Autodesk Fusion 360 part; units mm, degrees
(part 11 of 12)
  line L934 (66.0376, -20.82) -> (65.7437, -20.7245)
  line L935 (66.0427, -20.82) -> (66.0376, -20.82)
  line L936 (65.7437, -19.9155) -> (66.0376, -19.82)
  line L937 (66.5182, -20.4745) -> (66.3366, -20.7245)
  line L938 (65.5621, -20.1655) -> (65.7437, -19.9155)
  line L939 (66.5182, -20.1655) -> (66.5182, -20.4745)
  line L940 (66.0427, -19.82) -> (66.3366, -19.9155)
  line L941 (65.5621, -20.4745) -> (65.5621, -20.1655)
  line L942 (65.7437, -20.7245) -> (65.5621, -20.4745)
  line L943 (65.7437, -22.4555) -> (66.0376, -22.36)
  line L944 (66.3366, -22.4555) -> (66.5182, -22.7055)
  line L945 (66.5182, -23.0146) -> (66.3366, -23.2646)
  line L946 (66.0427, -22.36) -> (66.3366, -22.4555)
  line L947 (65.7437, -23.2646) -> (65.5621, -23.0146)
  line L948 (66.5182, -22.7055) -> (66.5182, -23.0146)
  line L949 (65.5621, -23.0146) -> (65.5621, -22.7055)
  line L950 (66.3366, -23.2646) -> (66.0427, -23.36)
  line L951 (66.0376, -23.36) -> (65.7437, -23.2646)
  line L952 (66.0427, -23.36) -> (66.0376, -23.36)
  line L953 (65.5621, -22.7055) -> (65.7437, -22.4555)
  line L954 (66.0376, -22.36) -> (66.0427, -22.36)
  line L955 (84.2982, -22.7055) -> (84.2982, -23.0146)
  line L956 (84.2982, -23.0146) -> (84.1166, -23.2646)
  line L957 (84.1166, -22.4555) -> (84.2982, -22.7055)
  line L958 (83.3421, -23.0146) -> (83.3421, -22.7055)
  line L959 (83.8227, -23.36) -> (83.8176, -23.36)
  line L960 (83.5237, -23.2646) -> (83.3421, -23.0146)
  line L961 (83.8227, -22.36) -> (84.1166, -22.4555)
  line L962 (83.8176, -23.36) -> (83.5237, -23.2646)
  line L963 (84.1166, -23.2646) -> (83.8227, -23.36)
  line L964 (83.5237, -22.4555) -> (83.8176, -22.36)
  line L965 (83.8176, -22.36) -> (83.8227, -22.36)
  line L966 (83.3421, -22.7055) -> (83.5237, -22.4555)
  line L967 (83.8176, -19.82) -> (83.8227, -19.82)
  line L968 (84.1166, -20.7245) -> (83.8227, -20.82)
  line L969 (83.8227, -19.82) -> (84.1166, -19.9155)
  line L970 (83.5237, -19.9155) -> (83.8176, -19.82)
  line L971 (84.1166, -19.9155) -> (84.2982, -20.1655)
  line L972 (84.2982, -20.4745) -> (84.1166, -20.7245)
  line L973 (83.3421, -20.4745) -> (83.3421, -20.1655)
  line L974 (84.2982, -20.1655) -> (84.2982, -20.4745)
  line L975 (83.5237, -20.7245) -> (83.3421, -20.4745)
  line L976 (83.8227, -20.82) -> (83.8176, -20.82)
  line L977 (83.8176, -20.82) -> (83.5237, -20.7245)
  line L978 (83.3421, -20.1655) -> (83.5237, -19.9155)
  line L979 (84.2982, -18.0062) -> (84.1166, -18.2562)
  line L980 (83.3421, -17.6972) -> (83.5237, -17.4472)
  line L981 (84.1166, -18.2562) -> (83.8227, -18.3517)
  line L982 (83.8227, -17.3517) -> (84.1166, -17.4472)
  line L983 (84.2982, -17.6972) -> (84.2982, -18.0062)
  line L984 (83.5237, -17.4472) -> (83.8176, -17.3517)
  line L985 (83.8176, -17.3517) -> (83.8227, -17.3517)
  line L986 (83.8227, -18.3517) -> (83.8176, -18.3517)
  line L987 (83.3421, -18.0062) -> (83.3421, -17.6972)
  line L988 (84.1166, -17.4472) -> (84.2982, -17.6972)
  line L989 (83.5237, -18.2562) -> (83.3421, -18.0062)
  line L990 (83.8176, -18.3517) -> (83.5237, -18.2562)
  line L991 (83.8176, -15.74) -> (83.5237, -15.6445)
  line L992 (84.2982, -15.0855) -> (84.2982, -15.3945)
  line L993 (83.8176, -14.74) -> (83.8227, -14.74)
  line L994 (83.8227, -14.74) -> (84.1166, -14.8355)
  line L995 (84.1166, -14.8355) -> (84.2982, -15.0855)
  line L996 (84.1166, -15.6445) -> (83.8227, -15.74)
  line L997 (84.2982, -15.3945) -> (84.1166, -15.6445)
  line L998 (83.3421, -15.0855) -> (83.5237, -14.8355)
  line L999 (83.5237, -15.6445) -> (83.3421, -15.3945)
  line L1000 (83.8227, -15.74) -> (83.8176, -15.74)
  line L1001 (83.3421, -15.3945) -> (83.3421, -15.0855)
  line L1002 (83.5237, -14.8355) -> (83.8176, -14.74)
  line L1003 (83.8176, -12.2) -> (83.8227, -12.2)
  line L1004 (83.5237, -12.2955) -> (83.8176, -12.2)
  line L1005 (83.8176, -13.2) -> (83.5237, -13.1045)
  line L1006 (84.1166, -13.1045) -> (83.8227, -13.2)
  line L1007 (83.8227, -13.2) -> (83.8176, -13.2)
  line L1008 (84.2982, -12.5455) -> (84.2982, -12.8545)
  line L1009 (83.8227, -12.2) -> (84.1166, -12.2955)
  line L1010 (84.1166, -12.2955) -> (84.2982, -12.5455)
  line L1011 (83.3421, -12.5455) -> (83.5237, -12.2955)
  line L1012 (84.2982, -12.8545) -> (84.1166, -13.1045)
  line L1013 (83.5237, -13.1045) -> (83.3421, -12.8545)
  line L1014 (83.3421, -12.8545) -> (83.3421, -12.5455)
  line L1015 (84.1166, -10.5645) -> (83.8227, -10.66)
  line L1016 (84.1166, -9.7555) -> (84.2982, -10.0055)
  line L1017 (83.8227, -9.66) -> (84.1166, -9.7555)
  line L1018 (83.5237, -9.7555) -> (83.8176, -9.66)
  line L1019 (84.2982, -10.0055) -> (84.2982, -10.3145)
  line L1020 (83.3421, -10.3145) -> (83.3421, -10.0055)
  line L1021 (83.8176, -9.66) -> (83.8227, -9.66)
  line L1022 (83.3421, -10.0055) -> (83.5237, -9.7555)
  line L1023 (83.8176, -10.66) -> (83.5237, -10.5645)
  line L1024 (83.5237, -10.5645) -> (83.3421, -10.3145)
  line L1025 (83.8227, -10.66) -> (83.8176, -10.66)
  line L1026 (84.2982, -10.3145) -> (84.1166, -10.5645)
  line L1027 (83.8176, -8.12) -> (83.5237, -8.0245)
  line L1028 (83.8227, -7.12) -> (84.1166, -7.2155)
  line L1029 (83.3421, -7.4655) -> (83.5237, -7.2155)
  line L1030 (83.8176, -7.12) -> (83.8227, -7.12)
  line L1031 (83.5237, -7.2155) -> (83.8176, -7.12)
  line L1032 (84.2982, -7.7745) -> (84.1166, -8.0245)
  line L1033 (83.8227, -8.12) -> (83.8176, -8.12)
  line L1034 (84.2982, -7.4655) -> (84.2982, -7.7745)
  line L1035 (83.3421, -7.7745) -> (83.3421, -7.4655)
  line L1036 (83.5237, -8.0245) -> (83.3421, -7.7745)
  line L1037 (84.1166, -7.2155) -> (84.2982, -7.4655)
  line L1038 (84.1166, -8.0245) -> (83.8227, -8.12)
  line L1039 (83.5237, -4.6755) -> (83.8176, -4.58)
  line L1040 (84.1166, -5.4845) -> (83.8227, -5.58)
  line L1041 (83.8227, -4.58) -> (84.1166, -4.6755)
  line L1042 (84.2982, -4.9255) -> (84.2982, -5.2345)
  line L1043 (84.1166, -4.6755) -> (84.2982, -4.9255)
  line L1044 (83.5237, -5.4845) -> (83.3421, -5.2345)
  line L1045 (83.3421, -5.2345) -> (83.3421, -4.9255)
  line L1046 (83.8176, -5.58) -> (83.5237, -5.4845)
  line L1047 (83.8176, -4.58) -> (83.8227, -4.58)
  line L1048 (83.3421, -4.9255) -> (83.5237, -4.6755)
  line L1049 (83.8227, -5.58) -> (83.8176, -5.58)
  line L1050 (84.2982, -5.2345) -> (84.1166, -5.4845)
  line L1051 (84.2982, -2.3855) -> (84.2982, -2.6945)
  line L1052 (83.5237, -2.1355) -> (83.8176, -2.04)
  line L1053 (83.5237, -2.9445) -> (83.3421, -2.6945)
  line L1054 (84.1166, -2.1355) -> (84.2982, -2.3855)
  line L1055 (83.8176, -2.04) -> (83.8227, -2.04)
  line L1056 (83.3421, -2.6945) -> (83.3421, -2.3855)
  line L1057 (83.8227, -2.04) -> (84.1166, -2.1355)
  line L1058 (83.8227, -3.04) -> (83.8176, -3.04)
  line L1059 (83.3421, -2.3855) -> (83.5237, -2.1355)
  line L1060 (83.8176, -3.04) -> (83.5237, -2.9445)
  line L1061 (84.1166, -2.9445) -> (83.8227, -3.04)
  line L1062 (84.2982, -2.6945) -> (84.1166, -2.9445)
  line L1063 (83.8176, -0.5) -> (83.5237, -0.4045)
  line L1064 (83.5237, 0.4045) -> (83.8176, 0.5)
  line L1065 (83.8176, 0.5) -> (83.8227, 0.5)
  line L1066 (83.5237, -0.4045) -> (83.3421, -0.1545)
  line L1067 (84.2982, 0.1545) -> (84.2982, -0.1545)
  line L1068 (84.1166, -0.4045) -> (83.8227, -0.5)
  line L1069 (83.3421, -0.1545) -> (83.3421, 0.1545)
  line L1070 (83.3421, 0.1545) -> (83.5237, 0.4045)
  line L1071 (83.8227, 0.5) -> (84.1166, 0.4045)
  line L1072 (83.8227, -0.5) -> (83.8176, -0.5)
  line L1073 (84.1166, 0.4045) -> (84.2982, 0.1545)
  line L1074 (84.2982, -0.1545) -> (84.1166, -0.4045)
  line L1075 (84.1166, 2.9445) -> (84.2982, 2.6945)
  line L1076 (83.5237, 2.1355) -> (83.3421, 2.3855)
  line L1077 (83.8227, 2.04) -> (83.8176, 2.04)
  line L1078 (84.2982, 2.6945) -> (84.2982, 2.3855)
  line L1079 (83.8227, 3.04) -> (84.1166, 2.9445)
  line L1080 (83.3421, 2.3855) -> (83.3421, 2.6945)
  line L1081 (83.8176, 3.04) -> (83.8227, 3.04)
  line L1082 (83.5237, 2.9445) -> (83.8176, 3.04)
  line L1083 (83.8176, 2.04) -> (83.5237, 2.1355)
  line L1084 (83.3421, 2.6945) -> (83.5237, 2.9445)
  line L1085 (84.2982, 2.3855) -> (84.1166, 2.1355)
  line L1086 (84.1166, 2.1355) -> (83.8227, 2.04)
  line L1087 (83.5237, 4.6755) -> (83.3421, 4.9255)
  line L1088 (83.3421, 4.9255) -> (83.3421, 5.2345)
  line L1089 (83.5237, 5.4845) -> (83.8176, 5.58)
  line L1090 (84.2982, 4.9255) -> (84.1166, 4.6755)
  line L1091 (83.8176, 5.58) -> (83.8227, 5.58)
  line L1092 (84.1166, 5.4845) -> (84.2982, 5.2345)
  line L1093 (84.1166, 4.6755) -> (83.8227, 4.58)
  line L1094 (83.3421, 5.2345) -> (83.5237, 5.4845)
  line L1095 (84.2982, 5.2345) -> (84.2982, 4.9255)
  line L1096 (83.8227, 5.58) -> (84.1166, 5.4845)
  line L1097 (83.8176, 4.58) -> (83.5237, 4.6755)
  line L1098 (83.8227, 4.58) -> (83.8176, 4.58)
  line L1099 (83.3421, 7.4655) -> (83.3421, 7.7745)
  line L1100 (83.3421, 7.7745) -> (83.5237, 8.0245)
  line L1101 (84.1166, 8.0245) -> (84.2982, 7.7745)
  line L1102 (83.5237, 8.0245) -> (83.8176, 8.12)
  line L1103 (83.8176, 7.12) -> (83.5237, 7.2155)
  line L1104 (84.2982, 7.4655) -> (84.1166, 7.2155)
  line L1105 (84.2982, 7.7745) -> (84.2982, 7.4655)
  line L1106 (83.5237, 7.2155) -> (83.3421, 7.4655)
  line L1107 (83.8176, 8.12) -> (83.8227, 8.12)
  line L1108 (83.8227, 8.12) -> (84.1166, 8.0245)
  line L1109 (83.8227, 7.12) -> (83.8176, 7.12)
  line L1110 (84.1166, 7.2155) -> (83.8227, 7.12)
  line L1111 (84.2982, 10.3145) -> (84.2982, 10.0055)
  line L1112 (83.8227, 10.66) -> (84.1166, 10.5645)
  line L1113 (83.8176, 10.66) -> (83.8227, 10.66)
  line L1114 (84.2982, 10.0055) -> (84.1166, 9.7555)
  line L1115 (83.3421, 10.0055) -> (83.3421, 10.3145)
  line L1116 (83.3421, 10.3145) -> (83.5237, 10.5645)
  line L1117 (83.8227, 9.66) -> (83.8176, 9.66)
  line L1118 (84.1166, 10.5645) -> (84.2982, 10.3145)
  line L1119 (83.5237, 9.7555) -> (83.3421, 10.0055)
  line L1120 (83.5237, 10.5645) -> (83.8176, 10.66)
  line L1121 (83.8176, 9.66) -> (83.5237, 9.7555)
  line L1122 (84.1166, 9.7555) -> (83.8227, 9.66)
  line L1123 (84.1166, 13.1045) -> (84.2982, 12.8545)
  line L1124 (83.3421, 12.8545) -> (83.5237, 13.1045)
  line L1125 (83.5237, 12.2955) -> (83.3421, 12.5455)
  line L1126 (83.8176, 12.2) -> (83.5237, 12.2955)
  line L1127 (83.3421, 12.5455) -> (83.3421, 12.8545)
  line L1128 (83.5237, 13.1045) -> (83.8176, 13.2)
  line L1129 (83.8227, 13.2) -> (84.1166, 13.1045)
  line L1130 (84.2982, 12.8545) -> (84.2982, 12.5455)
  line L1131 (84.1166, 12.2955) -> (83.8227, 12.2)
  line L1132 (84.2982, 12.5455) -> (84.1166, 12.2955)
  line L1133 (83.8176, 13.2) -> (83.8227, 13.2)
  line L1134 (83.8227, 12.2) -> (83.8176, 12.2)
  line L1135 (83.3421, 15.0855) -> (83.3421, 15.3945)
  line L1136 (83.5237, 15.6445) -> (83.8176, 15.74)
  line L1137 (83.5237, 14.8355) -> (83.3421, 15.0855)
  line L1138 (84.2982, 15.0855) -> (84.1166, 14.8355)
  line L1139 (83.3421, 15.3945) -> (83.5237, 15.6445)
  line L1140 (84.2982, 15.3945) -> (84.2982, 15.0855)
  line L1141 (84.1166, 15.6445) -> (84.2982, 15.3945)
  line L1142 (84.1166, 14.8355) -> (83.8227, 14.74)
  line L1143 (83.8176, 15.74) -> (83.8227, 15.74)
  line L1144 (83.8227, 14.74) -> (83.8176, 14.74)
  line L1145 (83.8176, 14.74) -> (83.5237, 14.8355)
  line L1146 (83.8227, 15.74) -> (84.1166, 15.6445)
  line L1147 (83.5237, 17.3755) -> (83.3421, 17.6255)
  line L1148 (83.8227, 18.28) -> (84.1166, 18.1845)
  line L1149 (83.3421, 17.9345) -> (83.5237, 18.1845)
  line L1150 (84.2982, 17.6255) -> (84.1166, 17.3755)
  line L1151 (83.8176, 17.28) -> (83.5237, 17.3755)
  line L1152 (84.2982, 17.9345) -> (84.2982, 17.6255)
  line L1153 (83.3421, 17.6255) -> (83.3421, 17.9345)
  line L1154 (84.1166, 18.1845) -> (84.2982, 17.9345)
  line L1155 (83.5237, 18.1845) -> (83.8176, 18.28)
  line L1156 (84.1166, 17.3755) -> (83.8227, 17.28)
  line L1157 (83.8227, 17.28) -> (83.8176, 17.28)
  line L1158 (83.8176, 18.28) -> (83.8227, 18.28)
  line L1159 (83.8227, 19.82) -> (83.8176, 19.82)
  line L1160 (83.5237, 20.7245) -> (83.8176, 20.82)
  line L1161 (83.3421, 20.4745) -> (83.5237, 20.7245)
  line L1162 (84.1166, 20.7245) -> (84.2982, 20.4745)
  line L1163 (84.2982, 20.4745) -> (84.2982, 20.1655)
  line L1164 (83.5237, 19.9155) -> (83.3421, 20.1655)
  line L1165 (83.8227, 20.82) -> (84.1166, 20.7245)
  line L1166 (84.2982, 20.1655) -> (84.1166, 19.9155)
  line L1167 (83.3421, 20.1655) -> (83.3421, 20.4745)
  line L1168 (83.8176, 20.82) -> (83.8227, 20.82)
  line L1169 (84.1166, 19.9155) -> (83.8227, 19.82)
  line L1170 (83.8176, 19.82) -> (83.5237, 19.9155)
  line L1171 (84.2982, 22.7055) -> (84.1166, 22.4555)
  line L1172 (83.5237, 23.2646) -> (83.8176, 23.36)
  line L1173 (83.8176, 22.36) -> (83.5237, 22.4555)
  line L1174 (84.1166, 23.2646) -> (84.2982, 23.0146)
  line L1175 (83.3421, 23.0146) -> (83.5237, 23.2646)
  line L1176 (84.2982, 23.0146) -> (84.2982, 22.7055)
  line L1177 (83.8227, 23.36) -> (84.1166, 23.2646)
  line L1178 (83.8227, 22.36) -> (83.8176, 22.36)
  line L1179 (83.3421, 22.7055) -> (83.3421, 23.0146)
  line L1180 (83.8176, 23.36) -> (83.8227, 23.36)
  line L1181 (84.1166, 22.4555) -> (83.8227, 22.36)
  line L1182 (83.5237, 22.4555) -> (83.3421, 22.7055)
  line L1183 (83.5237, 25.8046) -> (83.8176, 25.9001)
  line L1184 (84.1166, 24.9955) -> (83.8227, 24.9001)
  line L1185 (83.8227, 24.9001) -> (83.8176, 24.9001)
  line L1186 (84.1166, 25.8046) -> (84.2982, 25.5546)
  line L1187 (83.3421, 25.5546) -> (83.5237, 25.8046)
  line L1188 (83.8176, 25.9001) -> (83.8227, 25.9001)
  line L1189 (83.8227, 25.9001) -> (84.1166, 25.8046)
  line L1190 (84.2982, 25.5546) -> (84.2982, 25.2455)
  line L1191 (83.3421, 25.2455) -> (83.3421, 25.5546)
  line L1192 (84.2982, 25.2455) -> (84.1166, 24.9955)
  line L1193 (83.8176, 24.9001) -> (83.5237, 24.9955)
  line L1194 (83.5237, 24.9955) -> (83.3421, 25.2455)
  line L1195 (70.8237, -23.2646) -> (70.6421, -23.0146)
  line L1196 (71.1176, -23.36) -> (70.8237, -23.2646)
  line L1197 (71.5982, -23.0146) -> (71.4166, -23.2646)
  line L1198 (70.8237, -22.4555) -> (71.1176, -22.36)
  line L1199 (71.5982, -22.7055) -> (71.5982, -23.0146)
  line L1200 (71.4166, -23.2646) -> (71.1227, -23.36)
  line L1201 (71.1176, -22.36) -> (71.1227, -22.36)
  line L1202 (71.1227, -23.36) -> (71.1176, -23.36)
  line L1203 (70.6421, -23.0146) -> (70.6421, -22.7055)
  line L1204 (71.1227, -22.36) -> (71.4166, -22.4555)
  line L1205 (70.6421, -22.7055) -> (70.8237, -22.4555)
  line L1206 (71.4166, -22.4555) -> (71.5982, -22.7055)
  line L1207 (74.1382, -23.0146) -> (73.9566, -23.2646)
  line L1208 (73.1821, -22.7055) -> (73.3637, -22.4555)
  line L1209 (73.9566, -22.4555) -> (74.1382, -22.7055)
  line L1210 (73.1821, -23.0146) -> (73.1821, -22.7055)
  line L1211 (73.6627, -22.36) -> (73.9566, -22.4555)
  line L1212 (73.6576, -22.36) -> (73.6627, -22.36)
  line L1213 (73.6576, -23.36) -> (73.3637, -23.2646)
  line L1214 (73.3637, -22.4555) -> (73.6576, -22.36)
  line L1215 (74.1382, -22.7055) -> (74.1382, -23.0146)
  line L1216 (73.3637, -23.2646) -> (73.1821, -23.0146)
  line L1217 (73.6627, -23.36) -> (73.6576, -23.36)
  line L1218 (73.9566, -23.2646) -> (73.6627, -23.36)
  line L1219 (76.4966, -22.4555) -> (76.6782, -22.7055)
  line L1220 (76.6782, -23.0146) -> (76.4966, -23.2646)
  line L1221 (76.6782, -22.7055) -> (76.6782, -23.0146)
  line L1222 (76.4966, -23.2646) -> (76.2027, -23.36)
  line L1223 (76.2027, -22.36) -> (76.4966, -22.4555)
  line L1224 (76.2027, -23.36) -> (76.1976, -23.36)
  line L1225 (76.1976, -22.36) -> (76.2027, -22.36)
  line L1226 (75.9037, -22.4555) -> (76.1976, -22.36)
  line L1227 (75.7221, -22.7055) -> (75.9037, -22.4555)
  line L1228 (75.7221, -23.0146) -> (75.7221, -22.7055)
  line L1229 (75.9037, -23.2646) -> (75.7221, -23.0146)
  line L1230 (76.1976, -23.36) -> (75.9037, -23.2646)
  line L1231 (78.7376, -23.36) -> (78.4437, -23.2646)
  line L1232 (78.7376, -22.36) -> (78.7427, -22.36)
  line L1233 (79.0366, -23.2646) -> (78.7427, -23.36)
  line L1234 (79.2182, -23.0146) -> (79.0366, -23.2646)
  line L1235 (78.7427, -23.36) -> (78.7376, -23.36)
  line L1236 (79.2182, -22.7055) -> (79.2182, -23.0146)
  line L1237 (78.4437, -23.2646) -> (78.2621, -23.0146)
  line L1238 (78.7427, -22.36) -> (79.0366, -22.4555)
  line L1239 (79.0366, -22.4555) -> (79.2182, -22.7055)
  line L1240 (78.4437, -22.4555) -> (78.7376, -22.36)
  line L1241 (78.2621, -23.0146) -> (78.2621, -22.7055)
  line L1242 (78.2621, -22.7055) -> (78.4437, -22.4555)
  arc A2166 (-180.75, 30) -> (-179.25, 30) centre (-180, 30) ccw
  arc A2167 (-179.25, 30) -> (-180.75, 30) centre (-180, 30) ccw
  arc A2168 (-185.588, 27.46) -> (-187.112, 27.46) centre (-186.35, 27.46) ccw
  arc A2169 (-187.112, 27.46) -> (-185.588, 27.46) centre (-186.35, 27.46) ccw
  arc A2170 (-149.25, 30) -> (-150.75, 30) centre (-150, 30) ccw
  arc A2171 (-150.75, 30) -> (-149.25, 30) centre (-150, 30) ccw
  arc A2172 (-157.112, 27.46) -> (-155.588, 27.46) centre (-156.35, 27.46) ccw
  arc A2173 (-155.588, 27.46) -> (-157.112, 27.46) centre (-156.35, 27.46) ccw
  arc A2174 (-120.75, 30) -> (-119.25, 30) centre (-120, 30) ccw
  arc A2175 (-119.25, 30) -> (-120.75, 30) centre (-120, 30) ccw
  arc A2176 (-127.112, 27.46) -> (-125.588, 27.46) centre (-126.35, 27.46) ccw
  arc A2177 (-125.588, 27.46) -> (-127.112, 27.46) centre (-126.35, 27.46) ccw
  arc A2178 (-90.75, 30) -> (-89.25, 30) centre (-90, 30) ccw
  arc A2179 (-89.25, 30) -> (-90.75, 30) centre (-90, 30) ccw
  arc A2180 (-97.112, 27.46) -> (-95.588, 27.46) centre (-96.35, 27.46) ccw
  arc A2181 (-95.588, 27.46) -> (-97.112, 27.46) centre (-96.35, 27.46) ccw
  arc A2182 (-60.75, 30) -> (-59.25, 30) centre (-60, 30) ccw
  arc A2183 (-59.25, 30) -> (-60.75, 30) centre (-60, 30) ccw
  arc A2184 (-65.588, 27.46) -> (-67.112, 27.46) centre (-66.35, 27.46) ccw
  arc A2185 (-67.112, 27.46) -> (-65.588, 27.46) centre (-66.35, 27.46) ccw
  arc A2186 (-30.75, 30) -> (-29.25, 30) centre (-30, 30) ccw
  arc A2187 (-29.25, 30) -> (-30.75, 30) centre (-30, 30) ccw
  arc A2188 (-37.112, 27.46) -> (-35.588, 27.46) centre (-36.35, 27.46) ccw
  arc A2189 (-35.588, 27.46) -> (-37.112, 27.46) centre (-36.35, 27.46) ccw
  arc A2190 (-0.75, 30) -> (0.75, 30) centre (0, 30) ccw
  arc A2191 (0.75, 30) -> (-0.75, 30) centre (0, 30) ccw
  arc A2192 (-5.588, 27.46) -> (-7.112, 27.46) centre (-6.35, 27.46) ccw
  arc A2193 (-7.112, 27.46) -> (-5.588, 27.46) centre (-6.35, 27.46) ccw
  arc A2194 (29.25, 30) -> (30.75, 30) centre (30, 30) ccw
  arc A2195 (30.75, 30) -> (29.25, 30) centre (30, 30) ccw
  arc A2196 (24.412, 27.46) -> (22.888, 27.46) centre (23.65, 27.46) ccw
  arc A2197 (22.888, 27.46) -> (24.412, 27.46) centre (23.65, 27.46) ccw
  arc A2198 (-180.75, 0) -> (-179.25, 0) centre (-180, 0) ccw
  arc A2199 (-179.25, 0) -> (-180.75, 0) centre (-180, 0) ccw
  arc A2200 (-187.112, -2.54) -> (-185.588, -2.54) centre (-186.35, -2.54) ccw
  arc A2201 (-185.588, -2.54) -> (-187.112, -2.54) centre (-186.35, -2.54) ccw
  arc A2202 (-149.25, 0) -> (-150.75, 0) centre (-150, 0) ccw
  arc A2203 (-150.75, 0) -> (-149.25, 0) centre (-150, 0) ccw
  arc A2204 (-157.112, -2.54) -> (-155.588, -2.54) centre (-156.35, -2.54) ccw
  arc A2205 (-155.588, -2.54) -> (-157.112, -2.54) centre (-156.35, -2.54) ccw
  arc A2206 (-120.75, 0) -> (-119.25, 0) centre (-120, 0) ccw
  arc A2207 (-119.25, 0) -> (-120.75, 0) centre (-120, 0) ccw
  arc A2208 (-127.112, -2.54) -> (-125.588, -2.54) centre (-126.35, -2.54) ccw
  arc A2209 (-125.588, -2.54) -> (-127.112, -2.54) centre (-126.35, -2.54) ccw
  arc A2210 (-90.75, 0) -> (-89.25, 0) centre (-90, 0) ccw
  arc A2211 (-89.25, 0) -> (-90.75, 0) centre (-90, 0) ccw
  arc A2212 (-97.112, -2.54) -> (-95.588, -2.54) centre (-96.35, -2.54) ccw
  arc A2213 (-95.588, -2.54) -> (-97.112, -2.54) centre (-96.35, -2.54) ccw
  arc A2214 (-59.25, 0) -> (-60.75, 0) centre (-60, 0) ccw
  arc A2215 (-60.75, 0) -> (-59.25, 0) centre (-60, 0) ccw
  arc A2216 (-65.588, -2.54) -> (-67.112, -2.54) centre (-66.35, -2.54) ccw
  arc A2217 (-67.112, -2.54) -> (-65.588, -2.54) centre (-66.35, -2.54) ccw
  arc A2218 (-29.25, 0) -> (-30.75, 0) centre (-30, 0) ccw
  arc A2219 (-30.75, 0) -> (-29.25, 0) centre (-30, 0) ccw
  arc A2220 (-35.588, -2.54) -> (-37.112, -2.54) centre (-36.35, -2.54) ccw
  arc A2221 (-37.112, -2.54) -> (-35.588, -2.54) centre (-36.35, -2.54) ccw
  arc A2222 (13.601, -0.254) -> (15.101, -0.254) centre (14.351, -0.254) ccw
  arc A2223 (15.101, -0.254) -> (13.601, -0.254) centre (14.351, -0.254) ccw
  arc A2224 (7.239, -2.794) -> (8.763, -2.794) centre (8.001, -2.794) ccw
  line L1243 (8.763, -2.794) -> (8.763, -2.794)
  arc A2225 (8.763, -2.794) -> (7.239, -2.794) centre (8.001, -2.794) ccw
  arc A2226 (52.7171, -0.508) -> (54.2171, -0.508) centre (53.4671, -0.508) ccw
  arc A2227 (54.2171, -0.508) -> (52.7171, -0.508) centre (53.4671, -0.508) ccw
  arc A2228 (46.3551, -3.048) -> (47.8791, -3.048) centre (47.1171, -3.048) ccw
  arc A2229 (47.8791, -3.048) -> (46.3551, -3.048) centre (47.1171, -3.048) ccw
  arc A2230 (-191.47, -28.5751) -> (-192.97, -28.5751) centre (-192.22, -28.5751) ccw
  arc A2231 (-192.97, -28.5751) -> (-191.47, -28.5751) centre (-192.22, -28.5751) ccw
  arc A2232 (-197.808, -31.1151) -> (-199.332, -31.1151) centre (-198.57, -31.1151) ccw
  arc A2233 (-199.332, -31.1151) -> (-197.808, -31.1151) centre (-198.57, -31.1151) ccw
  arc A2234 (-162.97, -28.5751) -> (-161.47, -28.5751) centre (-162.22, -28.5751) ccw
  arc A2235 (-161.47, -28.5751) -> (-162.97, -28.5751) centre (-162.22, -28.5751) ccw
  arc A2236 (-169.332, -31.1151) -> (-167.808, -31.1151) centre (-168.57, -31.1151) ccw
  arc A2237 (-167.808, -31.1151) -> (-169.332, -31.1151) centre (-168.57, -31.1151) ccw
  arc A2238 (-132.97, -28.5751) -> (-131.47, -28.5751) centre (-132.22, -28.5751) ccw
  arc A2239 (-131.47, -28.5751) -> (-132.97, -28.5751) centre (-132.22, -28.5751) ccw
  arc A2240 (-137.808, -31.1151) -> (-139.332, -31.1151) centre (-138.57, -31.1151) ccw
  arc A2241 (-139.332, -31.1151) -> (-137.808, -31.1151) centre (-138.57, -31.1151) ccw
  arc A2242 (-102.97, -28.5751) -> (-101.47, -28.5751) centre (-102.22, -28.5751) ccw
  arc A2243 (-101.47, -28.5751) -> (-102.97, -28.5751) centre (-102.22, -28.5751) ccw
  arc A2244 (-109.332, -31.1151) -> (-107.808, -31.1151) centre (-108.57, -31.1151) ccw
  arc A2245 (-107.808, -31.1151) -> (-109.332, -31.1151) centre (-108.57, -31.1151) ccw
  arc A2246 (-71.47, -28.5751) -> (-72.97, -28.5751) centre (-72.22, -28.5751) ccw
  arc A2247 (-72.97, -28.5751) -> (-71.47, -28.5751) centre (-72.22, -28.5751) ccw
  arc A2248 (-79.332, -31.1151) -> (-77.808, -31.1151) centre (-78.57, -31.1151) ccw
  arc A2249 (-77.808, -31.1151) -> (-79.332, -31.1151) centre (-78.57, -31.1151) ccw
  arc A2250 (-41.47, -28.5751) -> (-42.97, -28.5751) centre (-42.22, -28.5751) ccw
  arc A2251 (-42.97, -28.5751) -> (-41.47, -28.5751) centre (-42.22, -28.5751) ccw
  arc A2252 (-49.332, -31.1151) -> (-47.808, -31.1151) centre (-48.57, -31.1151) ccw
  arc A2253 (-47.808, -31.1151) -> (-49.332, -31.1151) centre (-48.57, -31.1151) ccw
  arc A2254 (-11.47, -28.5751) -> (-12.97, -28.5751) centre (-12.22, -28.5751) ccw
  arc A2255 (-12.97, -28.5751) -> (-11.47, -28.5751) centre (-12.22, -28.5751) ccw
  arc A2256 (-19.332, -31.1151) -> (-17.808, -31.1151) centre (-18.57, -31.1151) ccw
  arc A2257 (-17.808, -31.1151) -> (-19.332, -31.1151) centre (-18.57, -31.1151) ccw
  arc A2258 (17.03, -28.5751) -> (18.53, -28.5751) centre (17.78, -28.5751) ccw
  arc A2259 (18.53, -28.5751) -> (17.03, -28.5751) centre (17.78, -28.5751) ccw
  arc A2260 (12.192, -31.1151) -> (10.668, -31.1151) centre (11.43, -31.1151) ccw
  arc A2261 (10.668, -31.1151) -> (12.192, -31.1151) centre (11.43, -31.1151) ccw
  arc A2262 (52.7146, -29.5911) -> (54.2146, -29.5911) centre (53.4646, -29.5911) ccw
  arc A2263 (54.2146, -29.5911) -> (52.7146, -29.5911) centre (53.4646, -29.5911) ccw
  arc A2264 (46.3526, -32.1311) -> (47.8766, -32.1311) centre (47.1146, -32.1311) ccw
  arc A2265 (47.8766, -32.1311) -> (46.3526, -32.1311) centre (47.1146, -32.1311) ccw
  arc A2266 (-186.1831, -55.6321) -> (-184.6831, -55.6321) centre (-185.4331, -55.6321) ccw
  arc A2267 (-184.6831, -55.6321) -> (-186.1831, -55.6321) centre (-185.4331, -55.6321) ccw
  arc A2268 (-192.5451, -58.1721) -> (-191.0211, -58.1721) centre (-191.7831, -58.1721) ccw
  arc A2269 (-191.0211, -58.1721) -> (-192.5451, -58.1721) centre (-191.7831, -58.1721) ccw
  arc A2270 (-156.1831, -55.6321) -> (-154.6831, -55.6321) centre (-155.4331, -55.6321) ccw
  arc A2271 (-154.6831, -55.6321) -> (-156.1831, -55.6321) centre (-155.4331, -55.6321) ccw
  arc A2272 (-162.5451, -58.1721) -> (-161.0211, -58.1721) centre (-161.7831, -58.1721) ccw
  arc A2273 (-161.0211, -58.1721) -> (-162.5451, -58.1721) centre (-161.7831, -58.1721) ccw
  arc A2274 (-126.1831, -55.6321) -> (-124.6831, -55.6321) centre (-125.4331, -55.6321) ccw
  arc A2275 (-124.6831, -55.6321) -> (-126.1831, -55.6321) centre (-125.4331, -55.6321) ccw
  arc A2276 (-131.0211, -58.1721) -> (-132.5451, -58.1721) centre (-131.7831, -58.1721) ccw
  arc A2277 (-132.5451, -58.1721) -> (-131.0211, -58.1721) centre (-131.7831, -58.1721) ccw
  arc A2278 (-96.1831, -55.6321) -> (-94.6831, -55.6321) centre (-95.4331, -55.6321) ccw
  arc A2279 (-94.6831, -55.6321) -> (-96.1831, -55.6321) centre (-95.4331, -55.6321) ccw
  arc A2280 (-102.5451, -58.1721) -> (-101.0211, -58.1721) centre (-101.7831, -58.1721) ccw
  arc A2281 (-101.0211, -58.1721) -> (-102.5451, -58.1721) centre (-101.7831, -58.1721) ccw
  arc A2282 (-66.1831, -55.6321) -> (-64.6831, -55.6321) centre (-65.4331, -55.6321) ccw
  arc A2283 (-64.6831, -55.6321) -> (-66.1831, -55.6321) centre (-65.4331, -55.6321) ccw
  arc A2284 (-72.5451, -58.1721) -> (-71.0211, -58.1721) centre (-71.7831, -58.1721) ccw
  arc A2285 (-71.0211, -58.1721) -> (-72.5451, -58.1721) centre (-71.7831, -58.1721) ccw
  arc A2286 (-36.1831, -55.6321) -> (-34.6831, -55.6321) centre (-35.4331, -55.6321) ccw
  arc A2287 (-34.6831, -55.6321) -> (-36.1831, -55.6321) centre (-35.4331, -55.6321) ccw
  arc A2288 (-41.0211, -58.1721) -> (-42.5451, -58.1721) centre (-41.7831, -58.1721) ccw
  arc A2289 (-42.5451, -58.1721) -> (-41.0211, -58.1721) centre (-41.7831, -58.1721) ccw
  arc A2290 (6.743, -56.6421) -> (8.243, -56.6421) centre (7.493, -56.6421) ccw
  arc A2291 (8.243, -56.6421) -> (6.743, -56.6421) centre (7.493, -56.6421) ccw
  arc A2292 (1.905, -59.1821) -> (0.381, -59.1821) centre (1.143, -59.1821) ccw
  arc A2293 (0.381, -59.1821) -> (1.905, -59.1821) centre (1.143, -59.1821) ccw
  arc A2294 (-174.9309, -86.7412) -> (-173.4309, -86.7412) centre (-174.1809, -86.7412) ccw
  arc A2295 (-173.4309, -86.7412) -> (-174.9309, -86.7412) centre (-174.1809, -86.7412) ccw
  arc A2296 (-181.2929, -89.2812) -> (-179.7689, -89.2812) centre (-180.5309, -89.2812) ccw
  arc A2297 (-179.7689, -89.2812) -> (-181.2929, -89.2812) centre (-180.5309, -89.2812) ccw
  arc A2298 (57.1381, -64.0081) -> (55.6381, -64.0081) centre (56.3881, -64.0081) ccw
  arc A2299 (55.6381, -64.0081) -> (57.1381, -64.0081) centre (56.3881, -64.0081) ccw
  arc A2300 (49.2761, -66.5481) -> (50.8001, -66.5481) centre (50.0381, -66.5481) ccw
  arc A2301 (50.8001, -66.5481) -> (49.2761, -66.5481) centre (50.0381, -66.5481) ccw
  arc A2302 (-144.5144, -86.7412) -> (-143.0144, -86.7412) centre (-143.7644, -86.7412) ccw
  arc A2303 (-143.0144, -86.7412) -> (-144.5144, -86.7412) centre (-143.7644, -86.7412) ccw
  arc A2304 (-149.3524, -89.2812) -> (-150.8764, -89.2812) centre (-150.1144, -89.2812) ccw
  arc A2305 (-150.8764, -89.2812) -> (-149.3524, -89.2812) centre (-150.1144, -89.2812) ccw
  arc A2306 (-112.5978, -86.7412) -> (-114.0978, -86.7412) centre (-113.3478, -86.7412) ccw
  arc A2307 (-114.0978, -86.7412) -> (-112.5978, -86.7412) centre (-113.3478, -86.7412) ccw
  arc A2308 (-120.4598, -89.2812) -> (-118.9358, -89.2812) centre (-119.6978, -89.2812) ccw
  arc A2309 (-118.9358, -89.2812) -> (-120.4598, -89.2812) centre (-119.6978, -89.2812) ccw
  arc A2310 (-82.1812, -86.7412) -> (-83.6812, -86.7412) centre (-82.9312, -86.7412) ccw
  arc A2311 (-83.6812, -86.7412) -> (-82.1812, -86.7412) centre (-82.9312, -86.7412) ccw
  arc A2312 (-88.5192, -89.2812) -> (-90.0432, -89.2812) centre (-89.2812, -89.2812) ccw
  arc A2313 (-90.0432, -89.2812) -> (-88.5192, -89.2812) centre (-89.2812, -89.2812) ccw
  arc A2314 (-51.7646, -86.7412) -> (-53.2647, -86.7412) centre (-52.5147, -86.7412) ccw
  arc A2315 (-53.2647, -86.7412) -> (-51.7646, -86.7412) centre (-52.5147, -86.7412) ccw
  arc A2316 (-58.1027, -89.2812) -> (-59.6267, -89.2812) centre (-58.8647, -89.2812) ccw
  arc A2317 (-59.6267, -89.2812) -> (-58.1027, -89.2812) centre (-58.8647, -89.2812) ccw
  arc A2318 (-22.8481, -86.7412) -> (-21.3481, -86.7412) centre (-22.0981, -86.7412) ccw
  arc A2319 (-21.3481, -86.7412) -> (-22.8481, -86.7412) centre (-22.0981, -86.7412) ccw
  arc A2320 (-29.2101, -89.2812) -> (-27.6861, -89.2812) centre (-28.4481, -89.2812) ccw
  arc A2321 (-27.6861, -89.2812) -> (-29.2101, -89.2812) centre (-28.4481, -89.2812) ccw
  arc A2322 (9.005, -86.8424) -> (7.505, -86.8424) centre (8.255, -86.8424) ccw
  arc A2323 (7.505, -86.8424) -> (9.005, -86.8424) centre (8.255, -86.8424) ccw
  arc A2324 (1.143, -89.3824) -> (2.667, -89.3824) centre (1.905, -89.3824) ccw
  arc A2325 (2.667, -89.3824) -> (1.143, -89.3824) centre (1.905, -89.3824) ccw
  arc A2326 (36.3911, -82.8042) -> (35.4911, -82.8042) centre (35.9411, -82.8042) ccw
  arc A2327 (35.4911, -82.8042) -> (36.3911, -82.8042) centre (35.9411, -82.8042) ccw
  arc A2328 (35.4911, -80.2642) -> (36.3911, -80.2642) centre (35.9411, -80.2642) ccw
  arc A2329 (36.3911, -80.2642) -> (35.4911, -80.2642) centre (35.9411, -80.2642) ccw
  arc A2330 (35.4911, -77.7242) -> (36.3911, -77.7242) centre (35.9411, -77.7242) ccw
  arc A2331 (36.3911, -77.7242) -> (35.4911, -77.7242) centre (35.9411, -77.7242) ccw
  arc A2332 (36.3911, -75.1842) -> (35.4911, -75.1842) centre (35.9411, -75.1842) ccw
  arc A2333 (35.4911, -75.1842) -> (36.3911, -75.1842) centre (35.9411, -75.1842) ccw
  arc A2334 (35.4911, -72.6441) -> (36.3911, -72.6441) centre (35.9411, -72.6441) ccw
  arc A2335 (36.3911, -72.6441) -> (35.4911, -72.6441) centre (35.9411, -72.6441) ccw
  arc A2336 (36.3911, -70.1041) -> (35.4911, -70.1041) centre (35.9411, -70.1041) ccw
  arc A2337 (35.4911, -70.1041) -> (36.3911, -70.1041) centre (35.9411, -70.1041) ccw
  arc A2338 (35.4911, -67.5641) -> (36.3911, -67.5641) centre (35.9411, -67.5641) ccw
  arc A2339 (36.3911, -67.5641) -> (35.4911, -67.5641) centre (35.9411, -67.5641) ccw
  arc A2340 (36.3911, -65.0241) -> (35.4911, -65.0241) centre (35.9411, -65.0241) ccw
  arc A2341 (35.4911, -65.0241) -> (36.3911, -65.0241) centre (35.9411, -65.0241) ccw
  arc A2342 (36.3911, -62.4841) -> (35.4911, -62.4841) centre (35.9411, -62.4841) ccw
  arc A2343 (35.4911, -62.4841) -> (36.3911, -62.4841) centre (35.9411, -62.4841) ccw
  arc A2344 (36.3911, -59.9441) -> (35.4911, -59.9441) centre (35.9411, -59.9441) ccw
  arc A2345 (35.4911, -59.9441) -> (36.3911, -59.9441) centre (35.9411, -59.9441) ccw
  arc A2346 (36.3911, -57.4041) -> (35.4911, -57.4041) centre (35.9411, -57.4041) ccw
  arc A2347 (35.4911, -57.4041) -> (36.3911, -57.4041) centre (35.9411, -57.4041) ccw
  arc A2348 (36.3911, -54.8641) -> (35.4911, -54.8641) centre (35.9411, -54.8641) ccw
  arc A2349 (35.4911, -54.8641) -> (36.3911, -54.8641) centre (35.9411, -54.8641) ccw
  arc A2350 (35.4911, -52.3241) -> (36.3911, -52.3241) centre (35.9411, -52.3241) ccw
  arc A2351 (36.3911, -52.3241) -> (35.4911, -52.3241) centre (35.9411, -52.3241) ccw
  arc A2352 (36.3911, -49.7841) -> (35.4911, -49.7841) centre (35.9411, -49.7841) ccw
  arc A2353 (35.4911, -49.7841) -> (36.3911, -49.7841) centre (35.9411, -49.7841) ccw
  arc A2354 (28.7711, -82.8042) -> (27.871, -82.8042) centre (28.3211, -82.8042) ccw
  arc A2355 (27.871, -82.8042) -> (28.7711, -82.8042) centre (28.3211, -82.8042) ccw
  arc A2356 (28.7711, -80.2642) -> (27.871, -80.2642) centre (28.3211, -80.2642) ccw
  arc A2357 (27.871, -80.2642) -> (28.7711, -80.2642) centre (28.3211, -80.2642) ccw
  arc A2358 (28.7711, -77.7242) -> (27.871, -77.7242) centre (28.3211, -77.7242) ccw
  arc A2359 (27.871, -77.7242) -> (28.7711, -77.7242) centre (28.3211, -77.7242) ccw
  arc A2360 (27.871, -75.1842) -> (28.7711, -75.1842) centre (28.3211, -75.1842) ccw
  arc A2361 (28.7711, -75.1842) -> (27.871, -75.1842) centre (28.3211, -75.1842) ccw
  arc A2362 (27.871, -72.6441) -> (28.7711, -72.6441) centre (28.3211, -72.6441) ccw
  arc A2363 (28.7711, -72.6441) -> (27.871, -72.6441) centre (28.3211, -72.6441) ccw
  arc A2364 (27.871, -70.1041) -> (28.7711, -70.1041) centre (28.3211, -70.1041) ccw
  arc A2365 (28.7711, -70.1041) -> (27.871, -70.1041) centre (28.3211, -70.1041) ccw
  arc A2366 (27.871, -67.5641) -> (28.7711, -67.5641) centre (28.3211, -67.5641) ccw
  arc A2367 (28.7711, -67.5641) -> (27.871, -67.5641) centre (28.3211, -67.5641) ccw
  arc A2368 (27.871, -65.0241) -> (28.7711, -65.0241) centre (28.3211, -65.0241) ccw
  arc A2369 (28.7711, -65.0241) -> (27.871, -65.0241) centre (28.3211, -65.0241) ccw
  arc A2370 (28.7711, -62.4841) -> (27.871, -62.4841) centre (28.3211, -62.4841) ccw
  arc A2371 (27.871, -62.4841) -> (28.7711, -62.4841) centre (28.3211, -62.4841) ccw
  arc A2372 (28.7711, -59.9441) -> (27.871, -59.9441) centre (28.3211, -59.9441) ccw
  arc A2373 (27.871, -59.9441) -> (28.7711, -59.9441) centre (28.3211, -59.9441) ccw
  arc A2374 (28.7711, -57.4041) -> (27.871, -57.4041) centre (28.3211, -57.4041) ccw
  arc A2375 (27.871, -57.4041) -> (28.7711, -57.4041) centre (28.3211, -57.4041) ccw
  arc A2376 (27.871, -54.8641) -> (28.7711, -54.8641) centre (28.3211, -54.8641) ccw
  arc A2377 (28.7711, -54.8641) -> (27.871, -54.8641) centre (28.3211, -54.8641) ccw
  arc A2378 (27.871, -52.3241) -> (28.7711, -52.3241) centre (28.3211, -52.3241) ccw
  arc A2379 (28.7711, -52.3241) -> (27.871, -52.3241) centre (28.3211, -52.3241) ccw
  arc A2380 (27.871, -49.7841) -> (28.7711, -49.7841) centre (28.3211, -49.7841) ccw
  arc A2381 (28.7711, -49.7841) -> (27.871, -49.7841) centre (28.3211, -49.7841) ccw
  arc A2382 (80.3332, -69.0881) -> (79.4331, -69.0881) centre (79.8832, -69.0881) ccw
  arc A2383 (79.4331, -69.0881) -> (80.3332, -69.0881) centre (79.8832, -69.0881) ccw
  arc A2384 (79.4331, -66.5481) -> (80.3332, -66.5481) centre (79.8832, -66.5481) ccw
  arc A2385 (80.3332, -66.5481) -> (79.4331, -66.5481) centre (79.8832, -66.5481) ccw
  arc A2386 (79.4331, -64.0081) -> (80.3332, -64.0081) centre (79.8832, -64.0081) ccw
  arc A2387 (80.3332, -64.0081) -> (79.4331, -64.0081) centre (79.8832, -64.0081) ccw
  arc A2388 (80.3332, -61.4681) -> (79.4331, -61.4681) centre (79.8832, -61.4681) ccw
  arc A2389 (79.4331, -61.4681) -> (80.3332, -61.4681) centre (79.8832, -61.4681) ccw
  arc A2390 (79.4331, -58.9281) -> (80.3332, -58.9281) centre (79.8832, -58.9281) ccw
  arc A2391 (80.3332, -58.9281) -> (79.4331, -58.9281) centre (79.8832, -58.9281) ccw
  arc A2392 (79.4331, -56.3881) -> (80.3332, -56.3881) centre (79.8832, -56.3881) ccw
  arc A2393 (80.3332, -56.3881) -> (79.4331, -56.3881) centre (79.8832, -56.3881) ccw
  arc A2394 (80.3332, -53.8481) -> (79.4331, -53.8481) centre (79.8832, -53.8481) ccw
  arc A2395 (79.4331, -53.8481) -> (80.3332, -53.8481) centre (79.8832, -53.8481) ccw
  arc A2396 (80.3332, -51.3081) -> (79.4331, -51.3081) centre (79.8832, -51.3081) ccw
  arc A2397 (79.4331, -51.3081) -> (80.3332, -51.3081) centre (79.8832, -51.3081) ccw
  arc A2398 (80.3332, -48.7681) -> (79.4331, -48.7681) centre (79.8832, -48.7681) ccw
  arc A2399 (79.4331, -48.7681) -> (80.3332, -48.7681) centre (79.8832, -48.7681) ccw
  arc A2400 (80.3332, -46.2281) -> (79.4331, -46.2281) centre (79.8832, -46.2281) ccw
  arc A2401 (79.4331, -46.2281) -> (80.3332, -46.2281) centre (79.8832, -46.2281) ccw
  arc A2402 (79.4331, -43.6881) -> (80.3332, -43.6881) centre (79.8832, -43.6881) ccw
  arc A2403 (80.3332, -43.6881) -> (79.4331, -43.6881) centre (79.8832, -43.6881) ccw
  arc A2404 (80.3332, -41.1481) -> (79.4331, -41.1481) centre (79.8832, -41.1481) ccw
  arc A2405 (79.4331, -41.1481) -> (80.3332, -41.1481) centre (79.8832, -41.1481) ccw
  arc A2406 (79.4331, -38.6081) -> (80.3332, -38.6081) centre (79.8832, -38.6081) ccw
  arc A2407 (80.3332, -38.6081) -> (79.4331, -38.6081) centre (79.8832, -38.6081) ccw
  arc A2408 (80.3332, -36.0681) -> (79.4331, -36.0681) centre (79.8832, -36.0681) ccw
  arc A2409 (79.4331, -36.0681) -> (80.3332, -36.0681) centre (79.8832, -36.0681) ccw
  arc A2410 (72.7132, -69.0881) -> (71.8131, -69.0881) centre (72.2631, -69.0881) ccw
  arc A2411 (71.8131, -69.0881) -> (72.7132, -69.0881) centre (72.2631, -69.0881) ccw
  arc A2412 (71.8131, -66.5481) -> (72.7132, -66.5481) centre (72.2631, -66.5481) ccw
  arc A2413 (72.7132, -66.5481) -> (71.8131, -66.5481) centre (72.2631, -66.5481) ccw
  arc A2414 (71.8131, -64.0081) -> (72.7132, -64.0081) centre (72.2631, -64.0081) ccw
  arc A2415 (72.7132, -64.0081) -> (71.8131, -64.0081) centre (72.2631, -64.0081) ccw
  arc A2416 (71.8131, -61.4681) -> (72.7132, -61.4681) centre (72.2631, -61.4681) ccw
  arc A2417 (72.7132, -61.4681) -> (71.8131, -61.4681) centre (72.2631, -61.4681) ccw
  arc A2418 (71.8131, -58.9281) -> (72.7132, -58.9281) centre (72.2631, -58.9281) ccw
  arc A2419 (72.7132, -58.9281) -> (71.8131, -58.9281) centre (72.2631, -58.9281) ccw
  arc A2420 (71.8131, -56.3881) -> (72.7132, -56.3881) centre (72.2631, -56.3881) ccw
  arc A2421 (72.7132, -56.3881) -> (71.8131, -56.3881) centre (72.2631, -56.3881) ccw
  arc A2422 (71.8131, -53.8481) -> (72.7132, -53.8481) centre (72.2631, -53.8481) ccw
  arc A2423 (72.7132, -53.8481) -> (71.8131, -53.8481) centre (72.2631, -53.8481) ccw
  arc A2424 (72.7132, -51.3081) -> (71.8131, -51.3081) centre (72.2631, -51.3081) ccw
  arc A2425 (71.8131, -51.3081) -> (72.7132, -51.3081) centre (72.2631, -51.3081) ccw
  arc A2426 (72.7132, -48.7681) -> (71.8131, -48.7681) centre (72.2631, -48.7681) ccw
  arc A2427 (71.8131, -48.7681) -> (72.7132, -48.7681) centre (72.2631, -48.7681) ccw
  arc A2428 (72.7132, -46.2281) -> (71.8131, -46.2281) centre (72.2631, -46.2281) ccw
  arc A2429 (71.8131, -46.2281) -> (72.7132, -46.2281) centre (72.2631, -46.2281) ccw
  arc A2430 (71.8131, -43.6881) -> (72.7132, -43.6881) centre (72.2631, -43.6881) ccw
  arc A2431 (72.7132, -43.6881) -> (71.8131, -43.6881) centre (72.2631, -43.6881) ccw
  arc A2432 (71.8131, -41.1481) -> (72.7132, -41.1481) centre (72.2631, -41.1481) ccw
  arc A2433 (72.7132, -41.1481) -> (71.8131, -41.1481) centre (72.2631, -41.1481) ccw
  arc A2434 (72.7132, -38.6081) -> (71.8131, -38.6081) centre (72.2631, -38.6081) ccw
  arc A2435 (71.8131, -38.6081) -> (72.7132, -38.6081) centre (72.2631, -38.6081) ccw
  arc A2436 (72.7132, -36.0681) -> (71.8131, -36.0681) centre (72.2631, -36.0681) ccw
  arc A2437 (71.8131, -36.0681) -> (72.7132, -36.0681) centre (72.2631, -36.0681) ccw
  arc A2438 (45.2811, -97.0282) -> (44.3811, -97.0282) centre (44.8311, -97.0282) ccw
  arc A2439 (44.3811, -97.0282) -> (45.2811, -97.0282) centre (44.8311, -97.0282) ccw
  arc A2440 (47.8211, -97.0282) -> (46.9211, -97.0282) centre (47.3711, -97.0282) ccw
  arc A2441 (46.9211, -97.0282) -> (47.8211, -97.0282) centre (47.3711, -97.0282) ccw
  arc A2442 (49.4611, -97.0282) -> (50.3611, -97.0282) centre (49.9111, -97.0282) ccw
  arc A2443 (50.3611, -97.0282) -> (49.4611, -97.0282) centre (49.9111, -97.0282) ccw
  arc A2444 (52.0011, -97.0282) -> (52.9011, -97.0282) centre (52.4511, -97.0282) ccw
  arc A2445 (52.9011, -97.0282) -> (52.0011, -97.0282) centre (52.4511, -97.0282) ccw
  arc A2446 (55.4411, -97.0282) -> (54.5411, -97.0282) centre (54.9911, -97.0282) ccw
  arc A2447 (54.5411, -97.0282) -> (55.4411, -97.0282) centre (54.9911, -97.0282) ccw
  arc A2448 (57.9811, -97.0282) -> (57.0811, -97.0282) centre (57.5311, -97.0282) ccw
  arc A2449 (57.0811, -97.0282) -> (57.9811, -97.0282) centre (57.5311, -97.0282) ccw
  arc A2450 (59.6211, -97.0282) -> (60.5211, -97.0282) centre (60.0711, -97.0282) ccw
  arc A2451 (60.5211, -97.0282) -> (59.6211, -97.0282) centre (60.0711, -97.0282) ccw
  arc A2452 (63.0611, -97.0282) -> (62.1611, -97.0282) centre (62.6111, -97.0282) ccw
  arc A2453 (62.1611, -97.0282) -> (63.0611, -97.0282) centre (62.6111, -97.0282) ccw
  arc A2454 (65.6011, -97.0282) -> (64.7011, -97.0282) centre (65.1511, -97.0282) ccw
  arc A2455 (64.7011, -97.0282) -> (65.6011, -97.0282) centre (65.1511, -97.0282) ccw
  arc A2456 (68.1411, -97.0282) -> (67.2411, -97.0282) centre (67.6911, -97.0282) ccw
  arc A2457 (67.2411, -97.0282) -> (68.1411, -97.0282) centre (67.6911, -97.0282) ccw
  arc A2458 (69.7811, -97.0282) -> (70.6812, -97.0282) centre (70.2311, -97.0282) ccw
  arc A2459 (70.6812, -97.0282) -> (69.7811, -97.0282) centre (70.2311, -97.0282) ccw
  arc A2460 (72.3211, -97.0282) -> (73.2212, -97.0282) centre (72.7711, -97.0282) ccw
  arc A2461 (73.2212, -97.0282) -> (72.3211, -97.0282) centre (72.7711, -97.0282) ccw
  arc A2462 (74.8611, -97.0282) -> (75.7612, -97.0282) centre (75.3112, -97.0282) ccw
  arc A2463 (75.7612, -97.0282) -> (74.8611, -97.0282) centre (75.3112, -97.0282) ccw
  arc A2464 (78.3012, -97.0282) -> (77.4011, -97.0282) centre (77.8512, -97.0282) ccw
  arc A2465 (77.4011, -97.0282) -> (78.3012, -97.0282) centre (77.8512, -97.0282) ccw
  arc A2466 (45.2811, -89.4082) -> (44.3811, -89.4082) centre (44.8311, -89.4082) ccw
  arc A2467 (44.3811, -89.4082) -> (45.2811, -89.4082) centre (44.8311, -89.4082) ccw
  arc A2468 (46.9211, -89.4082) -> (47.8211, -89.4082) centre (47.3711, -89.4082) ccw
  arc A2469 (47.8211, -89.4082) -> (46.9211, -89.4082) centre (47.3711, -89.4082) ccw
  arc A2470 (49.4611, -89.4082) -> (50.3611, -89.4082) centre (49.9111, -89.4082) ccw
  arc A2471 (50.3611, -89.4082) -> (49.4611, -89.4082) centre (49.9111, -89.4082) ccw
  arc A2472 (52.9011, -89.4082) -> (52.0011, -89.4082) centre (52.4511, -89.4082) ccw
  arc A2473 (52.0011, -89.4082) -> (52.9011, -89.4082) centre (52.4511, -89.4082) ccw
  arc A2474 (54.5411, -89.4082) -> (55.4411, -89.4082) centre (54.9911, -89.4082) ccw
  arc A2475 (55.4411, -89.4082) -> (54.5411, -89.4082) centre (54.9911, -89.4082) ccw
  arc A2476 (57.0811, -89.4082) -> (57.9811, -89.4082) centre (57.5311, -89.4082) ccw
  arc A2477 (57.9811, -89.4082) -> (57.0811, -89.4082) centre (57.5311, -89.4082) ccw
  arc A2478 (60.5211, -89.4082) -> (59.6211, -89.4082) centre (60.0711, -89.4082) ccw
  arc A2479 (59.6211, -89.4082) -> (60.5211, -89.4082) centre (60.0711, -89.4082) ccw
  arc A2480 (63.0611, -89.4082) -> (62.1611, -89.4082) centre (62.6111, -89.4082) ccw
  arc A2481 (62.1611, -89.4082) -> (63.0611, -89.4082) centre (62.6111, -89.4082) ccw
  arc A2482 (64.7011, -89.4082) -> (65.6011, -89.4082) centre (65.1511, -89.4082) ccw
  arc A2483 (65.6011, -89.4082) -> (64.7011, -89.4082) centre (65.1511, -89.4082) ccw
  arc A2484 (68.1411, -89.4082) -> (67.2411, -89.4082) centre (67.6911, -89.4082) ccw
  arc A2485 (67.2411, -89.4082) -> (68.1411, -89.4082) centre (67.6911, -89.4082) ccw
  arc A2486 (70.6812, -89.4082) -> (69.7811, -89.4082) centre (70.2311, -89.4082) ccw
  arc A2487 (69.7811, -89.4082) -> (70.6812, -89.4082) centre (70.2311, -89.4082) ccw
  arc A2488 (73.2212, -89.4082) -> (72.3211, -89.4082) centre (72.7711, -89.4082) ccw
  arc A2489 (72.3211, -89.4082) -> (73.2212, -89.4082) centre (72.7711, -89.4082) ccw
  arc A2490 (74.8611, -89.4082) -> (75.7612, -89.4082) centre (75.3112, -89.4082) ccw
  arc A2491 (75.7612, -89.4082) -> (74.8611, -89.4082) centre (75.3112, -89.4082) ccw
  arc A2492 (78.3012, -89.4082) -> (77.4011, -89.4082) centre (77.8512, -89.4082) ccw
  arc A2493 (77.4011, -89.4082) -> (78.3012, -89.4082) centre (77.8512, -89.4082) ccw
  arc A2494 (-155.4614, -117.1772) -> (-153.9613, -117.1772) centre (-154.7114, -117.1772) ccw
  arc A2495 (-153.9613, -117.1772) -> (-155.4614, -117.1772) centre (-154.7114, -117.1772) ccw
  arc A2496 (-161.8234, -119.7172) -> (-160.2994, -119.7172) centre (-161.0614, -119.7172) ccw
  arc A2497 (-160.2994, -119.7172) -> (-161.8234, -119.7172) centre (-161.0614, -119.7172) ccw
  arc A2498 (-111.302, -117.1772) -> (-112.802, -117.1772) centre (-112.052, -117.1772) ccw
  arc A2499 (-112.802, -117.1772) -> (-111.302, -117.1772) centre (-112.052, -117.1772) ccw
  arc A2500 (-119.164, -119.7172) -> (-117.64, -119.7172) centre (-118.402, -119.7172) ccw
  arc A2501 (-117.64, -119.7172) -> (-119.164, -119.7172) centre (-118.402, -119.7172) ccw
  arc A2502 (-82.802, -117.1772) -> (-81.302, -117.1772) centre (-82.052, -117.1772) ccw
  arc A2503 (-81.302, -117.1772) -> (-82.802, -117.1772) centre (-82.052, -117.1772) ccw
  arc A2504 (-87.64, -119.7172) -> (-89.164, -119.7172) centre (-88.402, -119.7172) ccw
  arc A2505 (-89.164, -119.7172) -> (-87.64, -119.7172) centre (-88.402, -119.7172) ccw
  arc A2506 (-52.802, -117.1772) -> (-51.302, -117.1772) centre (-52.052, -117.1772) ccw
  arc A2507 (-51.302, -117.1772) -> (-52.802, -117.1772) centre (-52.052, -117.1772) ccw
  arc A2508 (-57.64, -119.7172) -> (-59.164, -119.7172) centre (-58.402, -119.7172) ccw
  arc A2509 (-59.164, -119.7172) -> (-57.64, -119.7172) centre (-58.402, -119.7172) ccw
  arc A2510 (-21.302, -117.1772) -> (-22.802, -117.1772) centre (-22.052, -117.1772) ccw
  arc A2511 (-22.802, -117.1772) -> (-21.302, -117.1772) centre (-22.052, -117.1772) ccw
  arc A2512 (-29.164, -119.7172) -> (-27.64, -119.7172) centre (-28.402, -119.7172) ccw
  arc A2513 (-27.64, -119.7172) -> (-29.164, -119.7172) centre (-28.402, -119.7172) ccw
  arc A2514 (8.698, -117.1772) -> (7.198, -117.1772) centre (7.948, -117.1772) ccw
  arc A2515 (7.198, -117.1772) -> (8.698, -117.1772) centre (7.948, -117.1772) ccw
  arc A2516 (2.36, -119.7172) -> (0.836, -119.7172) centre (1.598, -119.7172) ccw
  arc A2517 (0.836, -119.7172) -> (2.36, -119.7172) centre (1.598, -119.7172) ccw
  arc A2518 (38.698, -117.1772) -> (37.198, -117.1772) centre (37.948, -117.1772) ccw
  arc A2519 (37.198, -117.1772) -> (38.698, -117.1772) centre (37.948, -117.1772) ccw
  arc A2520 (30.836, -119.7172) -> (32.36, -119.7172) centre (31.598, -119.7172) ccw
  arc A2521 (32.36, -119.7172) -> (30.836, -119.7172) centre (31.598, -119.7172) ccw
  line L1244 (-165.8504, 24.168) -> (-166.1285, 24.168)
  line L1245 (-165.6254, 25.7604) -> (-165.5394, 25.4959)
  line L1246 (-166.1285, 24.168) -> (-166.3535, 24.3315)
  line L1247 (-165.5394, 25.4959) -> (-165.5394, 24.596)
  line L1248 (-166.3535, 25.7604) -> (-166.1285, 25.9239)
  line L1249 (-165.5394, 24.596) -> (-165.6254, 24.3315)
  line L1250 (-166.4395, 24.596) -> (-166.4395, 25.4959)
  line L1251 (-165.8504, 25.9239) -> (-165.6254, 25.7604)
  line L1252 (-165.6254, 24.3315) -> (-165.8504, 24.168)
  line L1253 (-166.1285, 25.9239) -> (-165.8504, 25.9239)
  line L1254 (-166.3535, 24.3315) -> (-166.4395, 24.596)
  line L1255 (-166.4395, 25.4959) -> (-166.3535, 25.7604)
  line L1256 (-170.5378, 24.9243) -> (-170.2597, 24.9243)
  line L1257 (-170.0347, 24.7608) -> (-169.9488, 24.4963)
  line L1258 (-170.7628, 23.3316) -> (-170.8488, 23.5961)
  line L1259 (-170.2597, 24.9243) -> (-170.0347, 24.7608)
  line L1260 (-170.2597, 23.1682) -> (-170.5378, 23.1682)
  line L1261 (-170.0347, 23.3316) -> (-170.2597, 23.1682)
  line L1262 (-170.5378, 23.1682) -> (-170.7628, 23.3316)
  line L1263 (-169.9488, 23.5961) -> (-170.0347, 23.3316)
  line L1264 (-170.8488, 23.5961) -> (-170.8488, 24.4963)
  line L1265 (-170.8488, 24.4963) -> (-170.7628, 24.7608)
  line L1266 (-169.9488, 24.4963) -> (-169.9488, 23.5961)
  line L1267 (-170.7628, 24.7608) -> (-170.5378, 24.9243)
  line L1268 (-166.1285, 28.168) -> (-166.3535, 28.3315)
  line L1269 (-166.3535, 29.7604) -> (-166.1285, 29.9239)
  line L1270 (-166.3535, 28.3315) -> (-166.4395, 28.596)
  line L1271 (-165.5394, 29.4959) -> (-165.5394, 28.596)
  line L1272 (-165.5394, 28.596) -> (-165.6254, 28.3315)
  line L1273 (-165.6254, 28.3315) -> (-165.8504, 28.168)
  line L1274 (-165.8504, 28.168) -> (-166.1285, 28.168)
  line L1275 (-166.4395, 28.596) -> (-166.4395, 29.4959)
  line L1276 (-165.8504, 29.9239) -> (-165.6254, 29.7604)
  line L1277 (-166.4395, 29.4959) -> (-166.3535, 29.7604)
  line L1278 (-166.1285, 29.9239) -> (-165.8504, 29.9239)
  line L1279 (-165.6254, 29.7604) -> (-165.5394, 29.4959)
  line L1280 (-165.8503, 33.2631) -> (-165.6253, 33.0997)
  line L1281 (-166.4393, 31.935) -> (-166.4393, 32.8352)
  line L1282 (-166.1284, 31.507) -> (-166.3534, 31.6705)
  line L1283 (-165.5393, 31.935) -> (-165.6253, 31.6705)
  line L1284 (-165.8503, 31.507) -> (-166.1284, 31.507)
  line L1285 (-165.6253, 33.0997) -> (-165.5393, 32.8352)
  line L1286 (-166.3534, 33.0997) -> (-166.1284, 33.2631)
  line L1287 (-165.5393, 32.8352) -> (-165.5393, 31.935)
  line L1288 (-166.3534, 31.6705) -> (-166.4393, 31.935)
  line L1289 (-166.4393, 32.8352) -> (-166.3534, 33.0997)
  line L1290 (-165.6253, 31.6705) -> (-165.8503, 31.507)
  line L1291 (-166.1284, 33.2631) -> (-165.8503, 33.2631)
  arc A2522 (80.0128, -109.509) -> (79.7078, -109.509) centre (79.8603, -109.509) ccw
  arc A2523 (79.7078, -109.509) -> (80.0128, -109.509) centre (79.8603, -109.509) ccw
  arc A2524 (81.0796, -118.3868) -> (80.7746, -118.3868) centre (80.9271, -118.3868) ccw
  arc A2525 (80.7746, -118.3868) -> (81.0796, -118.3868) centre (80.9271, -118.3868) ccw
  arc A2526 (-137.2521, -37.6617) -> (-137.5571, -37.6617) centre (-137.4046, -37.6617) ccw
  arc A2527 (-137.5571, -37.6617) -> (-137.2521, -37.6617) centre (-137.4046, -37.6617) ccw
  arc A2528 (31.4904, -125.0968) -> (31.7954, -125.0968) centre (31.6429, -125.0968) ccw
  arc A2529 (31.7954, -125.0968) -> (31.4904, -125.0968) centre (31.6429, -125.0968) ccw
  arc A2530 (-96.1975, -5.6767) -> (-96.5025, -5.6767) centre (-96.35, -5.6767) ccw
  arc A2531 (-96.5025, -5.6767) -> (-96.1975, -5.6767) centre (-96.35, -5.6767) ccw